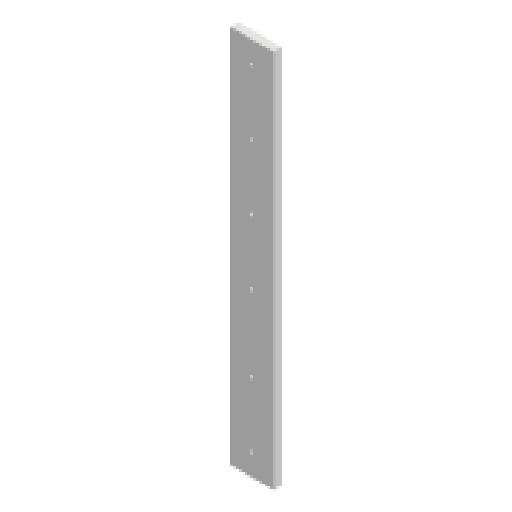
# Autodesk Inventor part: E
Saved by Autodesk Inventor 2024 (Build 280153000, 153)
## iProperties
Created: 2024-03-20
Part Number: E
Material: Generic
Document SubType Name: Modeling
Designer: marco
Density: 1 g/cm^3
Appearance: Wood - Painted White
Author: marco
Autodesk Inventor part; units mm, degrees
ref_plane "YZ Plane" through (0, 0, 0) normal (1, 0, 0) x (0, 1, 0)
ref_plane "XZ Plane" through (0, 0, 0) normal (0, 1, 0) x (-1, 0, 0)
ref_plane "XY Plane" through (0, 0, 0) normal (0, 0, 1) x (1, 0, 0)
sketch "Sketch1" plane through (0, 0, 0) normal (0, 0, 1) x (1, 0, 0)
  line L0 (-50, -437.5) -> (50, -437.5)
  line L1 (50, -437.5) -> (50, 437.5)
  line L2 (50, 437.5) -> (-50, 437.5)
  line L3 (-50, 437.5) -> (-50, -437.5)
  line L4 (-50, -437.5) -> (50, 437.5) construction
  line L5 (50, -437.5) -> (-50, 437.5) construction
  point P0 (0, 0)
  dimension "d0" = 100
  dimension "d1" = 875
  constraints: 12 end point, 2 midpoint, 2 parallel, 1 horizontal, 1 perpendicular
  measures "d0" distance of L2.end L1.end
  measures "d1" distance of L1.end L0.end
extrude "Extrusion1" add sketch "Sketch1" along normal mid plane 19
sketch "Sketch2" plane through (0, 0, 9.5) normal (0, 0, 1) x (1, 0, 0)
  line L0 (50, 437.5) -> (-50, 437.5) projected
  line L1 (0, 437.5) -> (0, 387.5)
  line L2 (0, 387.5) -> (0, 237.5)
  line L3 (0, 237.5) -> (0, 87.5)
  line L4 (0, 87.5) -> (0, -62.5)
  line L5 (0, -62.5) -> (0, -237.5)
  line L6 (0, -237.5) -> (0, -387.5)
  line L7 (0, -387.5) -> (0, -437.5)
  circle A0 centre (0, 387.5) radius 4
  circle A1 centre (0, 237.5) radius 4
  circle A2 centre (0, 87.5) radius 4
  circle A3 centre (0, -62.5) radius 4
  circle A4 centre (0, -237.5) radius 4
  circle A5 centre (0, -387.5) radius 4
  point P0 (0, 0)
  dimension "d4" = 50
  dimension "d5" = 150
  dimension "d6" = 150
  dimension "d7" = 150
  dimension "d8" = 175
  dimension "d9" = 150
  dimension "d10" = 50
  dimension "d11" = 8
  dimension "d12" = 8
  dimension "d13" = 8
  dimension "d14" = 8
  dimension "d15" = 8
  dimension "d16" = 8
  constraints: 14 end point, 6 centre point, 6 coincident, 4 point on line, 3 vertical, 1 midpoint
  measures "d4" distance of L1.start L1.end
  measures "d5" distance of L1.end L2.end
  measures "d6" distance of L2.end L3.end
  measures "d7" distance of L3.end L4.end
  measures "d8" distance of L4.end L5.end
  measures "d9" distance of L5.end L6.end
  measures "d10" distance of L6.end L7.end
  measures "d11" diameter of A0
  measures "d12" diameter of A1
  measures "d13" diameter of A2
  measures "d14" diameter of A3
  measures "d15" diameter of A4
  measures "d16" diameter of A5
extrude "Extrusion2" cut sketch "Sketch2" against normal through all
body "Solid1"
